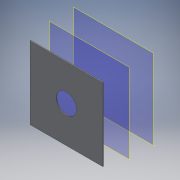
# Autodesk Inventor part: tapa_dummy
Saved by Autodesk Inventor 2019 (Build 230136000, 136)
## iProperties
Created: 2019-01-08
Part Number: tapa_dummy
Material: Generic
Document SubType Name: Modeling
Designer: jmc
Density: 1 g/cm^3
Appearance: Default
Author: jmc
Autodesk Inventor part; units mm, degrees
ref_plane "YZ Plane" through (0, 0, 0) normal (1, 0, 0) x (0, 1, 0)
ref_plane "XZ Plane" through (0, 0, 0) normal (0, 1, 0) x (-1, 0, 0)
ref_plane "XY Plane" through (0, 0, 0) normal (0, 0, 1) x (1, 0, 0)
ref_plane "Work Plane1" through (0, 0, 0) normal (0, 0, -1) x (-1, 0, 0)
sketch "Sketch1" plane through (0, 0, 0) normal (0, 0, -1) x (-1, 0, 0)
  line L0 (-115.3126, -90.0255) -> (64.6874, -90.0255)
  line L1 (64.6874, -90.0255) -> (64.6874, 89.9745)
  line L2 (64.6874, 89.9745) -> (-115.3126, 89.9745)
  line L3 (-115.3126, 89.9745) -> (-115.3126, -90.0255)
  line L4 (-25.3126, 0) -> (-25.3126, -88.1346) construction
  line L5 (-1.4905, -0.0255) -> (99.3864, -0.0255) construction
  point P0 (0, 0)
  point P1 (-25.3126, -0.0255)
  dimension "d0" = 180
  dimension "d1" = 180
  dimension "d8" = 90
  dimension "d9" = 90
  constraints: 12 end point, 2 parallel, 2 perpendicular, 1 horizontal, 1 vertical, 2 other
  measures "d0" distance of L2.end L1.end
  measures "d1" distance of L1.end L0.end
  measures "d8" distance from line of L2 point (-25.313, -0.026)
  measures "d9" distance from line of point (-25.313, -0.026) L1
extrude "Extrusion1" add sketch "Sketch1" along normal mid plane 2
sketch "Sketch2" plane through (0, 0, -1) normal (0, 0, -1) x (-1, 0, 0)
  circle A0 centre (-25, 0) radius 25.15 projected
  point P0 (0, 0)
extrude "Extrusion2" cut sketch "Sketch2" against normal through all
ref_plane "Work Plane3" through (0, 0, -56) normal (0, 0, -1) x (-1, 0, 0)
ref_plane "Work Plane2" through (0, 0, -116) normal (0, 0, -1) x (-1, 0, 0)
equation "\"d1\" = d0"
equation "\"d8\" = 0.5 * d0"
equation "\"d9\" = d8"
body "Solid1"
